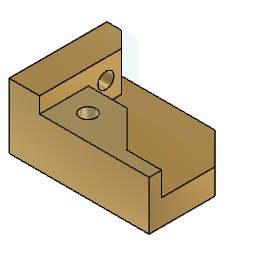
QUESTION 1 v1 (Autodesk Fusion 360 design; units mm, degrees)
Autodesk Fusion 360 part; units mm, degrees
sketch "Sketch1" plane through (0, 0, 0) normal (0, 0, 1) x (1, 0, 0)
  line L0 (88.0885, 61.5355) -> (-88.0885, 61.5355)
  line L1 (-88.0885, 61.5355) -> (-88.0885, -61.5355)
  line L2 (-88.0885, -61.5355) -> (88.0885, -61.5355)
  line L3 (88.0885, -61.5355) -> (88.0885, 61.5355)
  line L4 (88.0885, 61.5355) -> (-88.0885, -61.5355) construction
  line L5 (-88.0885, 61.5355) -> (88.0885, -61.5355) construction
  constraint horizontal L0
  constraint perpendicular L0 L1
  constraint parallel L0 L2
  constraint parallel L1 L3
  constraint coincident L4 origin
  constraint coincident L5 origin
extrude "Extrude1" add sketch "Sketch1" along normal blind 32
chamfer "Chamfer1" distance 40 angle 45 1 edges at (88.0885, 61.5355, 16)
sketch "Sketch2" plane through (0, 0, 32) normal (0, 0, 1) x (-1, 0, 0)
  line L0 (-88.0885, -21.5355) -> (-48.0885, -61.5355)
  line L1 (-48.0885, -61.5355) -> (88.0885, -61.5355)
  line L2 (88.0885, -61.5355) -> (88.0885, 61.5355)
  line L3 (88.0885, 61.5355) -> (-88.0885, 61.5355)
  line L4 (-88.0885, 61.5355) -> (-88.0885, -21.5355)
  line L5 (88.0885, 61.5355) -> (49.7061, 61.5355)
  line L6 (49.7061, 61.5355) -> (49.7061, -61.5355)
  line L7 (49.7061, -61.5355) -> (88.0885, -61.5355)
  line L8 (88.0885, -61.5355) -> (88.0885, 61.5355)
  constraint horizontal L5
  constraint vertical L6
  constraint horizontal L7
  constraint vertical L8
  constraint coincident L1 L6.end
  constraint coincident L2.end L3.start
extrude "Extrude2" add sketch "Sketch2" along normal blind 50 contours L1 L2 L3 L5 L6 L7 L8
sketch "Sketch3" plane through (0, 61.5355, 0) normal (0, 1, 0) x (-1, 0, 0)
  line L0 (-48.0885, 32) -> (-48.0885, 0)
  line L1 (-48.0885, 0) -> (88.0885, 0)
  line L2 (88.0885, 0) -> (88.0885, 82)
  line L3 (88.0885, 82) -> (49.7061, 82)
  line L4 (49.7061, 82) -> (49.7061, 32)
  line L5 (49.7061, 32) -> (-48.0885, 32)
chamfer "Chamfer2" distance 20 angle 45 1 edges at (-49.7061, 61.5355, 57)
sketch "Sketch4" plane through (0, 0, 32) normal (0, 0, 1) x (-1, 0, 0)
  line L0 (49.7061, -41.5355) -> (49.7061, 61.5355)
  line L1 (49.7061, 61.5355) -> (-88.0885, 61.5355)
  line L2 (-88.0885, 61.5355) -> (-88.0885, -21.5355)
  line L3 (-88.0885, -21.5355) -> (-48.0885, -61.5355)
  line L4 (-48.0885, -61.5355) -> (69.7061, -61.5355)
  line L5 (69.7061, -61.5355) -> (49.7061, -41.5355)
  line L6 (49.7061, 61.5355) -> (-43.9087, 61.5355)
  line L7 (-43.9087, 61.5355) -> (-43.9087, 0)
  line L8 (-43.9087, 0) -> (49.7061, 0)
  line L9 (49.7061, 0) -> (49.7061, 61.5355)
  constraint horizontal L6
  constraint vertical L7
  constraint horizontal L8
  constraint vertical L9
  constraint coincident L0.end L1.start
extrude "Extrude3" add sketch "Sketch4" along normal blind 30 contours L0 L1 L6 L7 L8 L9
chamfer "Chamfer3" distance 45 angle 45 1 edges at (43.9087, 0, 47)
sketch "Sketch5" plane through (0, 0, 32) normal (0, 0, 1) x (-1, 0, 0)
  line L0 (49.7061, 0) -> (1.0913, 0)
  line L1 (1.0913, 0) -> (-43.9087, 45)
  line L2 (-43.9087, 45) -> (-43.9087, 61.5355)
  line L3 (-43.9087, 61.5355) -> (-88.0885, 61.5355)
  line L4 (-88.0885, 61.5355) -> (-88.0885, -21.5355)
  line L5 (-88.0885, -21.5355) -> (-48.0885, -61.5355)
  line L6 (-48.0885, -61.5355) -> (69.7061, -61.5355)
  line L7 (69.7061, -61.5355) -> (49.7061, -41.5355)
  line L8 (49.7061, -41.5355) -> (49.7061, 0)
  line L9 (-43.9087, 61.5355) -> (-88.0885, 61.5355)
  line L10 (-88.0885, 61.5355) -> (-88.0885, 45.7382)
  line L11 (-88.0885, 45.7382) -> (-43.9087, 45.7382)
  line L12 (-43.9087, 45.7382) -> (-43.9087, 61.5355)
  constraint horizontal L9
  constraint vertical L10
  constraint horizontal L11
  constraint vertical L12
  constraint coincident L4 L10.end
  constraint coincident L2.end L3.start
extrude "Extrude4" add sketch "Sketch5" along normal blind 30 contours L2 L3 L4 L9 L10 L11 L12
sketch "Sketch6" plane through (0, 0, 62) normal (0, 0, 1) x (-1, 0, 0)
  line L0 (-43.9087, 45) -> (1.0913, 0)
  line L1 (1.0913, 0) -> (49.7061, 0)
  line L2 (49.7061, 0) -> (49.7061, 61.5355)
  line L3 (49.7061, 61.5355) -> (-88.0885, 61.5355)
  line L4 (-88.0885, 61.5355) -> (-88.0885, 45.7382)
  line L5 (-88.0885, 45.7382) -> (-43.9087, 45.7382)
  line L6 (-43.9087, 45.7382) -> (-43.9087, 45)
hole "Hole1" at (-49.7061, 21.9099, 57.0062) direction (-1, 0, 0) diameter 20 depth 0.01 tip angle 0.01
hole "Hole2" at (-20.3371, -30.0422, 62) direction (0, 0, -1) diameter 20 depth 0.01
hole "Hole3" at (-20.3371, -30.0422, 61.99) direction (0, 0, -1) diameter 20 depth 80
